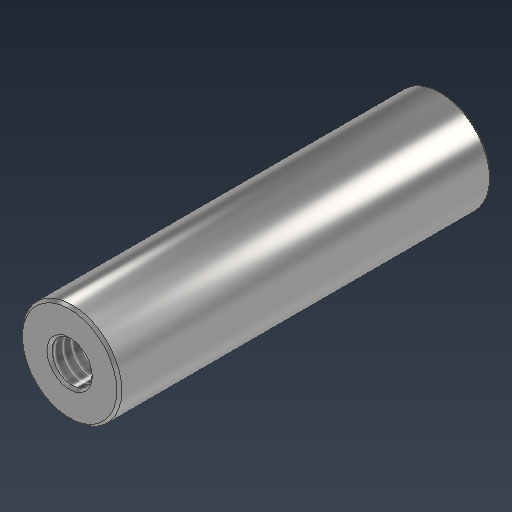
# Autodesk Inventor part: unir-spacer2
Saved by Autodesk Inventor 2021 (Build 250183000, 183)
## iProperties
Created: 2021-01-09
Part Number: unir-spacer2
Material: 鋼、炭素鋼
Document SubType Name: Modeling
Designer: Yuta Kage
Mass: 12.228 g
Surface Area: 12.1502 cm^2
Volume: 1.5577 cm^3
Density: 7.85 g/cm^3
Appearance: 半つや出し
Description: wilco
購入先: wilco
在庫数: 0.0
Author: Yuta Kage
Autodesk Inventor part; units mm, degrees
ref_plane "YZ Plane" through (0, 0, 0) normal (1, 0, 0) x (0, 1, 0)
ref_plane "XZ Plane" through (0, 0, 0) normal (0, 1, 0) x (-1, 0, 0)
ref_plane "XY Plane" through (0, 0, 0) normal (0, 0, 1) x (1, 0, 0)
sketch "スケッチ1" plane through (0, 0, 0) normal (0, 0, 1) x (1, 0, 0)
  circle A0 centre (0, 0) radius 4
  dimension "d13" = 8
  constraints: 1 centre point
  measures "d13" diameter of A0
extrude "押し出し1" add sketch "スケッチ1" along normal mid plane 30
sketch "スケッチ2" plane through (0, 0, 15) normal (0, 0, 1) x (1, 0, 0)
  point P0 (0, 0)
  point P1 (0, 0)
  constraints: 1 coincident
hole "穴1" at (0, 0, 15) direction (0, 0, -1) diameter 3.242 depth 11.8 tip angle 118 thread size "M4x0.7" class "6H" standard "ANSI Metric M Profile"
mirror "ミラー1" about plane through (0, 0, 0) normal (0, 0, 1) of "穴1"
chamfer "面取り1" distance 0.2 angle 45 4 edges at (0, 1.621, 15) (-4, 0, 15) (-4, 0, -15) (0, 1.621, -15)
